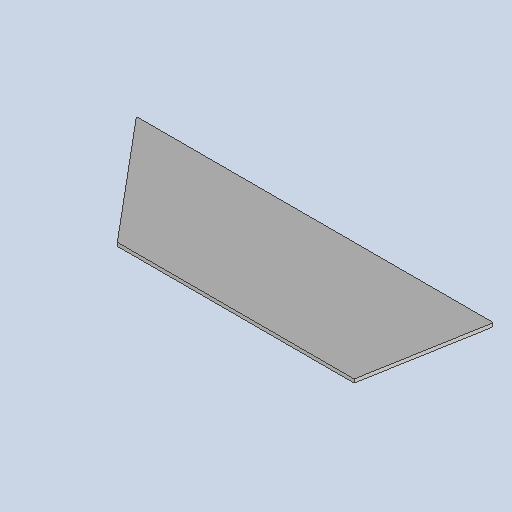
# Autodesk Inventor part: ДМФ 052 торец лотка кормовой v2.0
Saved by Autodesk Inventor 2026.2 (Build 302298000, 298)
## iProperties
Created: 2024-05-13
Part Number: ДМФ 052 торец лотка кормовой v2.0
Material: Generic
Document SubType Name: Sheet Metal
Designer: admin
Density: 1 g/cm^3
Sheet Metal Rule: Default
Appearance: Default
Mass: 40.1707 g
Surface Area: 283.602 cm^2
Volume: 40.1707 cm^3
Flat Pattern Width: 10 cm
Flat Pattern Length: 30.0726 cm
Flat Pattern Area: 300.726 cm^2
Sheet Metal Width: 100,000 mm
Sheet Metal Length: 300,726 mm
Sheet Metal Area: 30072,623 mm^2
Author: admin
Autodesk Inventor part; units mm, degrees
ref_plane "YZ Plane" through (0, 0, 0) normal (1, 0, 0) x (0, 1, 0)
ref_plane "XZ Plane" through (0, 0, 0) normal (0, 1, 0) x (-1, 0, 0)
ref_plane "XY Plane" through (0, 0, 0) normal (0, 0, 1) x (1, 0, 0)
sketch "Sketch1" plane through (0, 0, 0) normal (0, 0, 1) x (1, 0, 0)
  line L0 (-183.91, 100) -> (-100, 0)
  line L1 (-100, 0) -> (100, 0)
  line L2 (100, 0) -> (117.6327, 100)
  line L3 (117.6327, 100) -> (-183.91, 100)
  point P0 (0, 0)
  point P1 (0, 0)
  dimension "d0" = 100
  dimension "d1" = 200
  dimension "d2" = 301.5427
  dimension "d4" = 130
  dimension "d8" = 100
  measures "d0" distance between parallel lines of L1 L3
  measures "d1" distance of L0.end L1.end
  measures "d2" distance of L2.end L0.start
  measures "d4" angle of L1 L0
  measures "d8" angle of L1 L2
extrude "Plate1" add sketch "Sketch1" along normal blind 3
chamfer "Chamfer1" distance 1 angle 45 2 edges at (-183.91, 100, 1.5) (117.6327, 100, 1.5)
equation "\"d0\" = Лоток_высота"
equation "\"d4\" = Лоток_угол"
equation "\"d3\" = Thickness"
equation "\"BendRadius\" = Thickness"
equation "\"BendReliefWidth\" = Thickness"
equation "\"BendReliefDepth\" = 0.5 * Thickness"
equation "\"CornerReliefSize\" = 4 * Thickness"
equation "\"MinimumRemnant\" = 2 * Thickness"
equation "\"TransitionRadius\" = BendRadius"
equation "\"JacobiRadiusSize\" = BendRadius"
equation "\"GapSize\" = Thickness"
equation "\"Лоток_высота\" = 100"
equation "\"Лоток_угол\" = 130deg"
equation "\"Thickness\" = 3"
body "Solid1"
